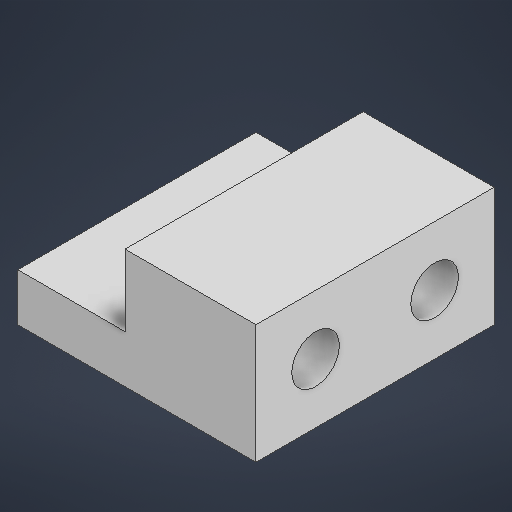
# Autodesk Inventor part: suport2_pcb_temp
Saved by Autodesk Inventor 2026.1 (Build 301233000, 233)
## iProperties
Created: 2025-09-26
Part Number: suport2_pcb_temp
Material: Generic
Document SubType Name: Modeling
Designer: emanuel
Density: 1 g/cm^3
Appearance: Default
Author: emanuel
Autodesk Inventor part; units mm, degrees
ref_plane "YZ Plane" through (0, 0, 0) normal (1, 0, 0) x (0, 1, 0)
ref_plane "XZ Plane" through (0, 0, 0) normal (0, 1, 0) x (-1, 0, 0)
ref_plane "XY Plane" through (0, 0, 0) normal (0, 0, 1) x (1, 0, 0)
sketch "Sketch1" plane through (0, 0, 0) normal (1, 0, 0) x (0, 1, 0)
  line L0 (0, 0) -> (5, 0)
  line L1 (5, 0) -> (5, -10)
  line L2 (5, -10) -> (0, -10)
  line L3 (0, -10) -> (0, 0)
  dimension "d0" = 5
  dimension "d1" = 10
  constraints: 8 end point, 2 parallel, 1 horizontal, 1 perpendicular
  measures "d0" distance of L1.end L2.end
  measures "d1" distance of L0.end L1.end
extrude "Extrusion1" add sketch "Sketch1" along normal blind 10
sketch "Sketch2" plane through (0, 5, 0) normal (0, 1, 0) x (1, 0, 0)
  line L0 (0, 0) -> (10, 0) projected
  line L1 (0, 10) -> (10, 10) projected
  line L2 (10, 0) -> (6.5, 0)
  line L3 (6.5, 0) -> (6.5, 10)
  line L4 (6.5, 10) -> (10, 10)
  line L5 (10, 10) -> (10, 0)
  line L6 (6.5, 0) -> (4.5, 0)
  line L7 (4.5, 0) -> (4.5, 10)
  line L8 (4.5, 10) -> (6.5, 10)
  line L9 (6.5, 10) -> (6.5, 0)
  line L10 (4.5, 10) -> (2, 10)
  line L11 (2, 10) -> (2, 0)
  line L12 (2, 0) -> (4.5, 0)
  line L13 (4.5, 0) -> (4.5, 10)
  line L14 (0, 10) -> (0, 0) projected
  line L15 (2, 0) -> (0, 0)
  line L16 (0, 0) -> (0, 10)
  line L17 (0, 10) -> (2, 10)
  line L18 (2, 10) -> (2, 0)
  dimension "d4" = 3.5
  dimension "d5" = 2
  dimension "d6" = 2.5
  constraints: 32 end point, 8 parallel, 4 horizontal, 4 perpendicular, 3 point on line
  measures "d4" distance of L3.end L4.end
  measures "d5" distance of L7.end L8.end
  measures "d6" distance of L12.end L11.end
extrude "Extrusion2" cut sketch "Sketch2" against normal blind 3 contours L14 L1 L11 L0 | L11 L1 L7 L0
sketch "Sketch3" plane through (10, 0, 0) normal (1, 0, 0) x (0, 0, -1)
  line L0 (10, 5) -> (0, 5) projected
  line L1 (0, 5) -> (2.5, 5)
  line L2 (2.5, 5) -> (2.5, 2.5)
  line L3 (2.5, 2.5) -> (0, 2.5)
  line L4 (0, 2.5) -> (0, 5)
  line L5 (10, 5) -> (7.5, 5)
  line L6 (7.5, 5) -> (7.5, 2.5)
  line L7 (7.5, 2.5) -> (10, 2.5)
  line L8 (10, 2.5) -> (10, 5)
  circle A0 centre (2.5, 2.5) radius 1
  circle A1 centre (7.5, 2.5) radius 1
  point P0 (0, 0)
  dimension "d9" = 2.5
  dimension "d10" = 2.5
  dimension "d11" = 2.5
  dimension "d12" = 2.5
  dimension "d13" = 2
  dimension "d14" = 2
  constraints: 16 end point, 4 parallel, 2 centre point, 2 coincident, 2 horizontal, 2 perpendicular
  measures "d9" distance of L2.end L3.end
  measures "d10" distance of L1.end L2.end
  measures "d11" distance of L7.end L6.end
  measures "d12" distance of L6.end L5.end
  measures "d13" diameter of A0
  measures "d14" diameter of A1
extrude "Extrusion3" cut sketch "Sketch3" against normal blind 5.5 contours A1 L7 L6 | L6 L7 A1 | A0 L3 L2 | L2 L3 A0
body "Solid1"
